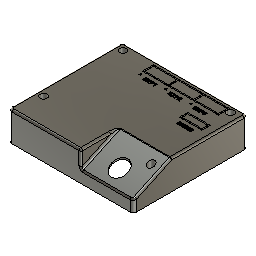
TFT35-E3-V3.0-case (Autodesk Fusion 360 design; units mm, degrees)
Autodesk Fusion 360 part; units mm, degrees
note: some values were not read from the file. Chosen so that the rebuilt part matches the saved one: which face or edge a step refers to; the layout of a text.
imported_body "Derived Base Feature1" makes body 1
move_body "Move1" bodies 1 to x (1, 0, 0) y (0, 0, 1) z (0, -1, 0) at (0, 0, 0)
sketch "mounting plate back" plane through (0, 0, 0) normal (0, 0, 1) x (-1, 0, 0)
  arc A0 (-83.1, -77.3055) -> (-80.1, -80.3055) centre (-80.1, -77.3055) ccw
  line L0 (-80.1, -80.3055) -> (15.9, -80.3055)
  arc A1 (15.9, -80.3055) -> (18.9, -77.3055) centre (15.9, -77.3055) ccw
  line L1 (18.9, -77.3055) -> (18.9, 33.4204)
  line L2 (18.9, 33.4204) -> (-83.1, 33.4204)
  line L3 (-83.1, 33.4204) -> (-83.1, -77.3055)
  line L4 (8.2, -16) -> (8.2, -68)
  line L5 (8.2, -68) -> (-71.6, -68)
  line L6 (-71.6, -68) -> (-71.6, -16)
  line L7 (-71.6, -16) -> (8.2, -16)
  circle A2 centre (0, 0) radius 5
  circle A3 centre (12.85, -9.55) radius 3
  circle A4 centre (12.85, -74.45) radius 3
  circle A5 centre (-75.05, -74.45) radius 3
  circle A6 centre (-75.05, -9.55) radius 3
  line L8 (18.9, 13) -> (-83.1, 13)
  line L9 (-83.1, 13) -> (-83.1, -80.2)
  line L10 (-83.1, -80.2) -> (18.9, -80.2)
  line L11 (18.9, -80.2) -> (18.9, 13)
  point P0 (12.85, -74.45)
  point P1 (-75.05, -74.45)
  point P2 (-75.05, -9.55)
  point P3 (12.85, -9.55)
  dimension "d5" = 93.2
  dimension "d6" = 102
  dimension "d7" = 13
  constraint coincident L1 L8.start
  constraint horizontal L8
  constraint vertical L9
  constraint horizontal L10
  constraint vertical L11
  constraint coincident P0 A4.centre
  constraint coincident P1 A5.centre
  constraint coincident P2 A6.centre
  constraint coincident P3 A3.centre
  constraint coincident A2.centre origin
  measures "d5" distance of L8.start L10.end
  measures "d6" distance of L8.start L8.end
  measures "d7" distance of L8 A2.centre
extrude "Extrude1" add sketch "mounting plate back" along normal blind 24 separate body contours A0 A1 L1 L3 L8 L9 L10 L11 | A0 L9 L10 | A1 L10 L11 | L4 L5 L6 L7 | A2 | A3 | A4 | A5 | A6 makes body 2
sketch "back box top" plane through (0, 0, 24) normal (0, 0, 1) x (-1, 0, 0)
  line L0 (18.9, -80.2) -> (18.9, 13)
  line L1 (18.9, 13) -> (-83.1, 13)
  line L2 (-83.1, 13) -> (-83.1, -80.2)
  line L3 (-83.1, -80.2) -> (18.9, -80.2)
  circle A0 centre (12.85, -74.45) radius 2.75
  circle A1 centre (-75.05, -74.45) radius 2.75
  circle A2 centre (12.85, -9.55) radius 2.75
  circle A3 centre (-75.05, -9.55) radius 2.75
  circle A4 centre (-59.9601, 1.1026) radius 6.75
  line L4 (-57.4705, -50.4562) -> (-75.7215, -50.4562)
  line L5 (-75.7215, -50.4562) -> (-75.7215, -57.1364)
  line L6 (-75.7215, -57.1364) -> (-57.4705, -57.1364)
  line L7 (-57.4705, -57.1364) -> (-57.4705, -50.4562)
  line L8 (-71.8313, -67.8197) -> (-9.744, -67.8197)
  line L9 (-9.744, -67.8197) -> (-9.744, -76.8684)
  line L10 (-9.744, -76.8684) -> (-71.8313, -76.8684)
  line L11 (-71.8313, -76.8684) -> (-71.8313, -67.8197)
  line L12 (-75.7215, -53.7963) -> (-57.4705, -53.7963) construction
  line L13 (-66.596, -50.4562) -> (-66.596, -57.1364) construction
  line L14 (-9.744, -72.3441) -> (-71.8313, -72.3441) construction
  line L15 (-74.7215, -56.1364) -> (-58.4705, -56.1364)
  line L16 (-58.4705, -56.1364) -> (-58.4705, -51.4562)
  line L17 (-58.4705, -51.4562) -> (-74.7215, -51.4562)
  line L18 (-74.7215, -51.4562) -> (-74.7215, -56.1364)
  line L19 (-65.596, -50.4562) -> (-67.596, -50.4562)
  line L20 (-67.596, -50.4562) -> (-67.596, -51.4562)
  line L21 (-65.596, -51.4562) -> (-65.596, -50.4562)
  line L22 (-57.4705, -54.7963) -> (-58.4705, -54.7963)
  line L23 (-58.4705, -52.7963) -> (-57.4705, -52.7963)
  line L24 (-57.4705, -52.7963) -> (-57.4705, -54.7963)
  line L25 (-67.596, -57.1364) -> (-65.596, -57.1364)
  line L26 (-65.596, -57.1364) -> (-65.596, -56.1364)
  line L27 (-67.596, -56.1364) -> (-67.596, -57.1364)
  line L28 (-75.7215, -54.7963) -> (-74.7215, -54.7963)
  line L29 (-74.7215, -52.7963) -> (-75.7215, -52.7963)
  line L30 (-75.7215, -52.7963) -> (-75.7215, -54.7963)
  line L31 (-70.8313, -75.8684) -> (-70.8313, -68.8197)
  line L32 (-10.744, -68.8197) -> (-10.744, -75.8684)
  line L33 (-71.8313, -73.3441) -> (-70.8313, -73.3441)
  line L34 (-70.8313, -71.3441) -> (-71.8313, -71.3441)
  line L35 (-71.8313, -71.3441) -> (-71.8313, -73.3441)
  line L36 (-9.744, -71.3441) -> (-10.744, -71.3441)
  line L37 (-10.744, -73.3441) -> (-9.744, -73.3441)
  line L38 (-9.744, -73.3441) -> (-9.744, -71.3441)
  line L39 (-40.7876, -76.8684) -> (-40.7876, -67.8197) construction
  line L40 (-39.7876, -67.8197) -> (-41.7876, -67.8197)
  line L41 (-41.7876, -67.8197) -> (-41.7876, -68.8197)
  line L42 (-39.7876, -68.8197) -> (-39.7876, -67.8197)
  line L43 (-41.7876, -76.8684) -> (-39.7876, -76.8684)
  line L44 (-39.7876, -76.8684) -> (-39.7876, -75.8684)
  line L45 (-41.7876, -75.8684) -> (-41.7876, -76.8684)
  line L46 (-30.4396, -67.8197) -> (-30.4396, -76.8684) construction
  line L47 (-51.1356, -67.8197) -> (-51.1356, -76.8684) construction
  line L48 (-29.9396, -68.8197) -> (-29.9396, -75.8684)
  line L49 (-30.9396, -75.8684) -> (-30.9396, -68.8197)
  line L50 (-29.9396, -68.8197) -> (-10.744, -68.8197)
  line L51 (-10.744, -75.8684) -> (-29.9396, -75.8684)
  line L52 (-30.9396, -73.3441) -> (-30.4396, -73.3441)
  line L53 (-20.3418, -68.8197) -> (-20.3418, -75.8684) construction
  line L54 (-19.3418, -67.8197) -> (-21.3418, -67.8197)
  line L55 (-21.3418, -67.8197) -> (-21.3418, -68.8197)
  line L56 (-19.3418, -68.8197) -> (-19.3418, -67.8197)
  line L57 (-21.3418, -76.8684) -> (-21.3418, -75.8684)
  line L58 (-19.3418, -75.8684) -> (-19.3418, -76.8684)
  line L59 (-50.6356, -75.8684) -> (-50.6356, -68.8197)
  line L60 (-51.6356, -68.8197) -> (-51.6356, -75.8684)
  line L61 (-70.8313, -68.8197) -> (-51.6356, -68.8197)
  line L62 (-50.6356, -68.8197) -> (-30.9396, -68.8197)
  line L63 (-30.9396, -75.8684) -> (-50.6356, -75.8684)
  line L64 (-51.6356, -75.8684) -> (-70.8313, -75.8684)
  line L65 (-51.6356, -73.3441) -> (-50.6356, -73.3441)
  line L66 (-50.6356, -73.3441) -> (-50.6356, -71.3441)
  line L67 (-50.6356, -71.3441) -> (-51.6356, -71.3441)
  line L68 (-51.6356, -71.3441) -> (-51.6356, -73.3441)
  line L69 (-61.2335, -68.8197) -> (-61.2335, -75.8684) construction
  line L70 (-60.2335, -67.8197) -> (-62.2335, -67.8197)
  line L71 (-62.2335, -67.8197) -> (-62.2335, -68.8197)
  line L72 (-60.2335, -68.8197) -> (-60.2335, -67.8197)
  line L73 (-62.2335, -76.8684) -> (-60.2335, -76.8684)
  line L74 (-60.2335, -76.8684) -> (-60.2335, -75.8684)
  line L75 (-62.2335, -75.8684) -> (-62.2335, -76.8684)
  line L76 (-30.9396, -73.3441) -> (-29.9396, -73.3441)
  line L77 (-29.9396, -73.3441) -> (-29.9396, -71.3441)
  line L78 (-29.9396, -71.3441) -> (-30.9396, -71.3441)
  line L79 (-30.9396, -71.3441) -> (-30.9396, -73.3441)
  line L80 (-30.9396, -73.3441) -> (-29.9396, -71.3441) construction
  line L81 (-29.9396, -73.3441) -> (-30.9396, -71.3441) construction
  line L82 (-52.2335, -76.8684) -> (-52.2335, -75.8684)
  line L83 (-54.2335, -75.8684) -> (-54.2335, -76.8684)
  line L84 (-54.2335, -76.8684) -> (-52.2335, -76.8684)
  line L85 (-68.2335, -76.8684) -> (-68.2335, -75.8684)
  line L86 (-70.2335, -75.8684) -> (-70.2335, -76.8684)
  line L87 (-70.2335, -76.8684) -> (-68.2335, -76.8684)
  line L88 (-54.2335, -67.8197) -> (-54.2335, -68.8197)
  line L89 (-52.2335, -67.8197) -> (-54.2335, -67.8197)
  line L90 (-52.2335, -68.8197) -> (-52.2335, -67.8197)
  line L91 (-70.2335, -67.8197) -> (-70.2335, -68.8197)
  line L92 (-68.2335, -67.8197) -> (-70.2335, -67.8197)
  line L93 (-68.2335, -68.8197) -> (-68.2335, -67.8197)
  line L94 (-33.7876, -76.8684) -> (-31.7876, -76.8684)
  line L95 (-31.7876, -76.8684) -> (-31.7876, -75.8684)
  line L96 (-33.7876, -75.8684) -> (-33.7876, -76.8684)
  line L97 (-49.7876, -76.8684) -> (-47.7876, -76.8684)
  line L98 (-47.7876, -76.8684) -> (-47.7876, -75.8684)
  line L99 (-49.7876, -75.8684) -> (-49.7876, -76.8684)
  line L100 (-31.7876, -68.8197) -> (-31.7876, -67.8197)
  line L101 (-31.7876, -67.8197) -> (-33.7876, -67.8197)
  line L102 (-33.7876, -67.8197) -> (-33.7876, -68.8197)
  line L103 (-47.7876, -68.8197) -> (-47.7876, -67.8197)
  line L104 (-47.7876, -67.8197) -> (-49.7876, -67.8197)
  line L105 (-49.7876, -67.8197) -> (-49.7876, -68.8197)
  line L106 (-11.3418, -68.8197) -> (-11.3418, -67.8197)
  line L107 (-11.3418, -67.8197) -> (-13.3418, -67.8197)
  line L108 (-13.3418, -67.8197) -> (-13.3418, -68.8197)
  line L109 (-27.3418, -68.8197) -> (-27.3418, -67.8197)
  line L110 (-27.3418, -67.8197) -> (-29.3418, -67.8197)
  line L111 (-29.3418, -67.8197) -> (-29.3418, -68.8197)
  line L112 (-21.3418, -76.8684) -> (-21.3418, -75.8684)
  line L113 (-19.3418, -75.8684) -> (-19.3418, -76.8684)
  line L114 (-11.3418, -75.8684) -> (-11.3418, -76.8684)
  line L115 (-11.3418, -75.8684) -> (-11.3418, -76.8684)
  line L116 (-13.3418, -76.8684) -> (-13.3418, -75.8684)
  line L117 (-13.3418, -76.8684) -> (-13.3418, -75.8684)
  line L118 (-27.3418, -75.8684) -> (-27.3418, -76.8684)
  line L119 (-27.3418, -75.8684) -> (-27.3418, -76.8684)
  line L120 (-29.3418, -76.8684) -> (-29.3418, -75.8684)
  line L121 (-29.3418, -76.8684) -> (-29.3418, -75.8684)
  line L122 (-61.096, -56.1364) -> (-61.096, -57.1364)
  line L123 (-59.096, -57.1364) -> (-59.096, -56.1364)
  line L124 (-61.096, -57.1364) -> (-59.096, -57.1364)
  line L125 (-73.996, -56.1364) -> (-73.996, -57.1364)
  line L126 (-71.996, -57.1364) -> (-71.996, -56.1364)
  line L127 (-73.996, -57.1364) -> (-71.996, -57.1364)
  line L128 (-72.096, -51.4562) -> (-72.096, -50.4562)
  line L129 (-74.096, -50.4562) -> (-74.096, -51.4562)
  line L130 (-72.096, -50.4562) -> (-74.096, -50.4562)
  line L131 (-59.096, -51.4562) -> (-59.096, -50.4562)
  line L132 (-61.096, -50.4562) -> (-61.096, -51.4562)
  line L133 (-59.096, -50.4562) -> (-61.096, -50.4562)
  line L134 (-9.9786, -61.8197) -> (-71.9086, -61.8197) construction
  line L135 (-57.8501, -44.4562) -> (-75.3418, -44.4562) construction
  line L136 (-66.596, -50.4562) -> (-66.596, -44.4562) construction
  line L137 (-61.2335, -68.8197) -> (-61.2335, -61.8197) construction
  line L138 (-40.7876, -68.8197) -> (-40.7876, -61.8197) construction
  line L139 (-20.3418, -68.8197) -> (-20.3418, -61.8197) construction
  line L140 (-15.6983, -61.8197) -> (-24.9854, -61.8197) construction
  line L141 (-24.9854, -61.8197) -> (-24.9854, -65.8197) construction
  line L142 (-24.9854, -65.8197) -> (-15.6983, -65.8197) construction
  line L143 (-15.6983, -65.8197) -> (-15.6983, -61.8197) construction
  line L144 (-35.9195, -61.8197) -> (-45.6558, -61.8197) construction
  line L145 (-45.6558, -61.8197) -> (-45.6558, -65.8197) construction
  line L146 (-45.6558, -65.8197) -> (-35.9195, -65.8197) construction
  line L147 (-35.9195, -65.8197) -> (-35.9195, -61.8197) construction
  line L148 (-56.3507, -61.8197) -> (-66.1163, -61.8197) construction
  line L149 (-66.1163, -61.8197) -> (-66.1163, -65.8197) construction
  line L150 (-66.1163, -65.8197) -> (-56.3507, -65.8197) construction
  line L151 (-56.3507, -65.8197) -> (-56.3507, -61.8197) construction
  line L152 (-60.7278, -44.4562) -> (-72.4642, -44.4562) construction
  line L153 (-72.4642, -44.4562) -> (-72.4642, -48.4562) construction
  line L154 (-72.4642, -48.4562) -> (-60.7278, -48.4562) construction
  line L155 (-60.7278, -48.4562) -> (-60.7278, -44.4562) construction
  line L156 (-12.2078, -64.0824) -> (-11.3418, -65.5824)
  line L157 (-11.3418, -65.5824) -> (-10.4758, -64.0824)
  line L158 (-10.4758, -64.0824) -> (-12.2078, -64.0824)
  line L159 (-12.2078, -64.0824) -> (-11.3418, -65.5824)
  line L160 (-11.3418, -65.5824) -> (-10.4758, -64.0824)
  line L161 (-10.4758, -64.0824) -> (-12.2078, -64.0824)
  line L162 (-32.9038, -64.0824) -> (-32.0378, -65.5824)
  line L163 (-32.0378, -65.5824) -> (-31.1718, -64.0824)
  line L164 (-32.9038, -64.0824) -> (-32.0378, -65.5824)
  line L165 (-31.1718, -64.0824) -> (-32.9038, -64.0824)
  line L166 (-32.0378, -65.5824) -> (-31.1718, -64.0824)
  line L167 (-31.1718, -64.0824) -> (-32.9038, -64.0824)
  line L168 (-53.5998, -64.0824) -> (-52.7338, -65.5824)
  line L169 (-51.8678, -64.0824) -> (-53.5998, -64.0824)
  line L170 (-53.5998, -64.0824) -> (-52.7338, -65.5824)
  line L171 (-51.8678, -64.0824) -> (-53.5998, -64.0824)
  line L172 (-52.7338, -65.5824) -> (-51.8678, -64.0824)
  line L173 (-52.7338, -65.5824) -> (-51.8678, -64.0824)
  point P0 (12.85, -74.45)
  point P1 (-75.05, -74.45)
  point P2 (-75.05, -9.55)
  point P3 (12.85, -9.55)
  point P4 (-30.4396, -72.3441)
  point P5 (-20.3418, -68.8197)
  point P6 (-20.3418, -75.8684)
  point P7 (-51.1356, -72.3441)
  point P8 (-61.2335, -68.8197)
  point P9 (-61.2335, -75.8684)
  point P10 (-30.4396, -72.3441)
  point P11 (-53.2335, -75.8684)
  point P12 (-53.2335, -75.8684)
  point P13 (-69.2335, -75.8684)
  point P14 (-69.2335, -75.8684)
  point P15 (-53.2335, -68.8197)
  point P16 (-53.2335, -68.8197)
  point P17 (-69.2335, -68.8197)
  point P18 (-69.2335, -68.8197)
  point P19 (-32.7876, -76.8684)
  point P20 (-48.7876, -76.8684)
  point P21 (-32.7876, -67.8197)
  point P22 (-48.7876, -67.8197)
  point P23 (-12.3418, -68.8197)
  point P24 (-12.3418, -68.8197)
  point P25 (-28.3418, -68.8197)
  point P26 (-28.3418, -68.8197)
  point P27 (-20.3418, -75.8684)
  point P28 (-20.3418, -75.8684)
  point P29 (-12.3418, -75.8684)
  point P30 (-12.3418, -75.8684)
  point P31 (-12.3418, -75.8684)
  point P32 (-12.3418, -75.8684)
  point P33 (-28.3418, -75.8684)
  point P34 (-28.3418, -75.8684)
  point P35 (-28.3418, -75.8684)
  point P36 (-28.3418, -75.8684)
  point P37 (-60.096, -57.1364)
  point P38 (-72.996, -57.1364)
  point P39 (-73.096, -50.4562)
  point P40 (-60.096, -50.4562)
  point P41 (-11.3418, -64.5824)
  point P42 (-11.3418, -64.5824)
  point P43 (-32.0378, -64.5824)
  point P44 (-32.0378, -64.5824)
  point P45 (-52.7338, -64.5824)
  point P46 (-52.7338, -64.5824)
  dimension "d21" = 5.5
  dimension "d22" = 5.5
  dimension "d23" = 5.5
  dimension "d24" = 5.5
  dimension "d37" = 13.5
  dimension "d101" = -1
  dimension "d118" = 20.6957
  dimension "d119" = 20.6957
  dimension "d120" = 1
  dimension "d125" = 1
  dimension "d126" = 2
  dimension "d141" = 6
  dimension "d142" = 6
  dimension "d146" = 0.5
  dimension "d147" = 0.5
  dimension "d148" = 0.5
  dimension "d149" = 0.5
  dimension "d150" = 0.5
  dimension "d151" = 0.5
  text T0 "EXP1" font "Arial" height 4 bold align ink ink in box 0 x 0 at (-15.7083, -61.8397) x (-1, 0) y (0, -1) spacing 1 height is em
  text T1 "EXP2" font "Arial" height 4 bold align ink ink in box 0 x 0 at (-35.9295, -61.8397) x (-1, 0) y (0, -1) spacing 1 height is em
  text T2 "EXP3" font "Arial" height 4 bold align ink ink in box 0 x 0 at (-56.3607, -61.8397) x (-1, 0) y (0, -1) spacing 1 height is em
  text T3 "RS232" font "Arial" height 4 bold align ink ink in box 0 x 0 at (-60.7378, -44.4762) x (-1, 0) y (0, -1) spacing 1 height is em
  constraint coincident P0 A0.centre
  constraint coincident P1 A1.centre
  constraint coincident P3 A2.centre
  constraint coincident P2 A3.centre
  constraint midpoint L4 L13.start
  constraint perpendicular L19 L20
  constraint parallel L20 L21
  constraint horizontal L19
  constraint coincident L4 L19.start
  constraint parallel L22 L23
  constraint horizontal L22
  constraint perpendicular L25 L26
  constraint parallel L26 L27
  constraint horizontal L25
  constraint parallel L28 L29
  constraint horizontal L28
  constraint parallel L33 L34
  constraint horizontal L33
  constraint parallel L36 L37
  constraint horizontal L36
  constraint parallel L11 L31
  constraint parallel L8 L61
  constraint parallel L9 L32
  constraint perpendicular L40 L41
  constraint parallel L41 L42
  constraint horizontal L40
  constraint perpendicular L43 L44
  constraint parallel L44 L45
  constraint horizontal L43
  constraint coincident L8 L46.start
  constraint coincident L10 L46.end
  constraint perpendicular L10 L46
  constraint coincident L8 L47.start
  constraint coincident L10 L47.end
  constraint perpendicular L10 L47
  constraint parallel L48 L49
  constraint collinear L50 L61
  constraint collinear L51 L63
  constraint horizontal L52
  constraint midpoint L50 P5
  constraint midpoint L51 P28
  constraint perpendicular L51 L53
  constraint perpendicular L54 L55
  constraint parallel L55 L56
  constraint horizontal L54
  constraint coincident P5 L53.start
  constraint parallel L57 L58
  constraint coincident P28 P27
  constraint parallel L59 L60
  constraint collinear L61 L62
  constraint collinear L63 L64
  constraint perpendicular L65 L66
  constraint parallel L65 L67
  constraint parallel L66 L68
  constraint horizontal L65
  constraint midpoint L61 P8
  constraint midpoint L64 P9
  constraint perpendicular L64 L69
  constraint perpendicular L70 L71
  constraint parallel L71 L72
  constraint horizontal L70
  constraint coincident P8 L69.start
  constraint perpendicular L73 L74
  constraint parallel L74 L75
  constraint horizontal L73
  constraint coincident P9 L69.end
  constraint coincident L64 L74.end
  constraint coincident L64 L75.start
  constraint coincident L31 L33.end
  constraint coincident L31 L34.start
  constraint coincident L61 L71.end
  constraint coincident L61 L72.start
  constraint coincident L63 L45.start
  constraint coincident L63 L44.end
  constraint coincident L62 L41.end
  constraint coincident L62 L42.start
  constraint coincident L49 L52.start
  constraint coincident L46 L52.end
  constraint perpendicular L76 L77
  constraint parallel L76 L78
  constraint parallel L77 L79
  constraint horizontal L76
  constraint coincident L80 P10
  constraint coincident L81 P10
  constraint coincident P10 P4
  constraint coincident L50 L56.start
  constraint coincident L50 L55.end
  constraint coincident L51 L58.start
  constraint coincident L51 L57.end
  constraint coincident L10 L57.start
  constraint coincident L10 L58.end
  constraint coincident L32 L37.start
  constraint coincident L32 L36.end
  constraint coincident L18 L29.start
  constraint coincident L18 L28.end
  constraint coincident L15 L27.start
  constraint coincident L15 L26.end
  constraint coincident L17 L20.end
  constraint coincident L17 L21.start
  constraint coincident L16 L23.start
  constraint coincident L16 L22.end
  constraint perpendicular L82 L84
  constraint parallel L82 L83
  constraint horizontal L84
  constraint coincident P12 P11
  constraint perpendicular L85 L87
  constraint parallel L85 L86
  constraint horizontal L87
  constraint coincident P14 P13
  constraint perpendicular L88 L89
  constraint parallel L88 L90
  constraint horizontal L89
  constraint coincident P16 P15
  constraint perpendicular L91 L92
  constraint parallel L91 L93
  constraint horizontal L92
  constraint coincident P18 P17
  constraint perpendicular L94 L95
  constraint parallel L95 L96
  constraint horizontal L94
  constraint perpendicular L97 L98
  constraint parallel L98 L99
  constraint horizontal L97
  constraint perpendicular L101 L102
  constraint parallel L100 L102
  constraint horizontal L101
  constraint perpendicular L104 L105
  constraint parallel L103 L105
  constraint horizontal L104
  constraint perpendicular L107 L108
  constraint parallel L106 L108
  constraint horizontal L107
  constraint coincident P24 P23
  constraint perpendicular L110 L111
  constraint parallel L109 L111
  constraint horizontal L110
  constraint coincident P26 P25
  constraint parallel L112 L113
  constraint parallel L114 L117
  constraint coincident P32 P31
  constraint parallel L115 L116
  constraint parallel L118 L121
  constraint coincident P36 P35
  constraint parallel L119 L120
  constraint perpendicular L123 L124
  constraint parallel L122 L123
  constraint horizontal L124
  constraint perpendicular L126 L127
  constraint parallel L125 L126
  constraint horizontal L127
  constraint perpendicular L129 L130
  constraint parallel L128 L129
  constraint horizontal L130
  constraint perpendicular L132 L133
  constraint parallel L131 L132
  constraint horizontal L133
  constraint horizontal L134
  constraint perpendicular L131 L135
  constraint midpoint L135 L136.end
  constraint vertical L13
  constraint vertical L136
  constraint coincident L134 L137.end
  constraint perpendicular L134 L137
  constraint midpoint L62 L138.start
  constraint coincident L134 L138.end
  constraint perpendicular L134 L138
  constraint coincident L134 L139.end
  constraint perpendicular L134 L139
  constraint perpendicular L140 L141
  constraint parallel L140 L142
  constraint parallel L141 L143
  constraint perpendicular L144 L145
  constraint parallel L144 L146
  constraint parallel L145 L147
  constraint midpoint L138.end L144
  constraint perpendicular L148 L149
  constraint parallel L148 L150
  constraint parallel L149 L151
  constraint perpendicular L152 L153
  constraint parallel L152 L154
  constraint parallel L153 L155
  measures "d21" diameter of A0
  measures "d22" diameter of A1
  measures "d23" diameter of A2
  measures "d24" diameter of A3
  measures "d37" diameter of A4
  measures "d118" distance of L9 L46
  measures "d119" distance of L11 L47
  measures "d120" distance of L48.end L49.start
  measures "d125" distance of L59.end L60.start
  measures "d126" distance of L65.end L66.end
  measures "d141" distance of L8 L134
  measures "d142" distance of L4 L135
  measures "d146" distance of P42 L158
  measures "d147" distance of P42 L161
  measures "d148" distance of P44 L167
  measures "d149" distance of P44 L165
  measures "d150" distance of P46 L169
  measures "d151" distance of P46 L171
sketch "inside bracket face" plane through (0, -27.4513, -12.8008) normal (0, 0.906308, 0.422618) x (-1, 0, 0)
  arc A0 (-80.1, 57.1241) -> (-83.1, 54.1241) centre (-80.1, 54.1241) ccw
  line L0 (-83.1, 54.1241) -> (-83.1, 14.1241)
  line L1 (-83.1, 14.1241) -> (18.9, 14.1241)
  line L2 (18.9, 14.1241) -> (18.9, 54.1241)
  arc A1 (18.9, 54.1241) -> (15.9, 57.1241) centre (15.9, 54.1241) ccw
  line L3 (15.9, 57.1241) -> (-80.1, 57.1241)
  circle A2 centre (-73.1, 48.1241) radius 2.8
  circle A3 centre (-53.1, 28.1241) radius 2.8
  line L4 (-83.1, 14.1241) -> (-40.1, 14.1241)
  line L5 (-40.1, 14.1241) -> (-40.1, 57.1241)
  line L6 (-40.1, 57.1241) -> (-83.1, 57.1241)
  line L7 (-83.1, 57.1241) -> (-83.1, 14.1241)
  dimension "d28" = 43
  constraint horizontal L4
  constraint vertical L5
  constraint horizontal L6
  constraint vertical L7
  constraint coincident L0.end L1.start
  measures "d28" distance of L0.end L4.end
extrude "Extrude4" cut sketch "inside bracket face" along normal blind 120 contours A0 L0 L1 L3 L4 L5 L6 L7 | A0 L6 L7 | A2 | A3 bodies 2
extrude "Extrude3" cut sketch "back box top" against normal blind 12.75 contours A0 | A1 | A2 | A3 bodies 2
move_face "OffsetFaces2" offset -0.1 4 faces at (-15.5966, 9.6871, 15.5) (-15.515, 75.1286, 15.5) (72.385, 75.1286, 15.5) (72.3035, 9.4105, 17.0435) on bodies 2
fillet "Fillet2" radius 2.75 4 edges at (-18.9, 80.2, 12) (83.1, 80.2, 12) (83.1, -13, 4.7611) (-18.9, -13, 12) on bodies 2
fillet "Fillet2" radius 1.5 10 edges at (83.1, 49.1239, 24) (61.6, 18.0478, 24) (83.1, 2.5239, 16.7611) (40.1, 2.5239, 16.7611) (40.1, 2.5239, 24) (40.1, -13, 16.7611) (10.6, -13, 24) (61.6, -13, 9.5222) (-18.9, 33.6, 24) (32.1, 80.2, 24) on bodies 2
shell "Shell2" thickness 1.25 removed faces 1 at (16.0167, 49.1333, 0) on bodies 2
hole "Hole1" at (-12.85, 74.45, 24) at (75.05, 74.45, 24) at (75.05, 9.55, 24) at (-12.85, 9.55, 24) direction (0, 0, -1) diameter 3.2 depth 15 tip angle 180 bodies 2
sketch "inside back box" plane through (0, 0, 22.75) normal (0, 0, -1) x (1, 0, 0)
  ellipse E0 centre (41.6, -11.2817) end of major axis (41.6, -18.3803) minor radius 3 (38.6, -11.2817) -> (41.6, -18.3803) ccw
  line L0 (38.6, -11.2817) -> (38.6, 11.5)
  line L1 (38.6, 11.5) -> (-16.15, 11.5)
  arc A0 (-16.15, 11.5) -> (-17.4, 10.25) centre (-16.15, 10.25) ccw
  line L2 (-17.4, 10.25) -> (-17.4, -77.45)
  arc A1 (-17.4, -77.45) -> (-16.15, -78.7) centre (-16.15, -77.45) ccw
  line L3 (-16.15, -78.7) -> (80.35, -78.7)
  arc A2 (80.35, -78.7) -> (81.6, -77.45) centre (80.35, -77.45) ccw
  line L4 (81.6, -77.45) -> (81.6, -18.3803)
  line L5 (81.6, -18.3803) -> (41.6, -18.3803)
  circle A3 centre (-12.85, -9.55) radius 4.1
  circle A4 centre (75.05, -74.45) radius 4.1
  circle A5 centre (-12.85, -74.45) radius 4.1
  line L6 (-16.15, 10.25) -> (23.85, 10.25)
  line L7 (23.85, 10.25) -> (23.85, -8.75)
  line L8 (23.85, -8.75) -> (-16.15, -8.75)
  line L9 (-16.15, -8.75) -> (-16.15, 10.25)
  dimension "d156" = 1.25
  dimension "d157" = 40
  dimension "d158" = 19
  constraint horizontal L6
  constraint vertical L7
  constraint horizontal L8
  constraint vertical L9
  constraint coincident A0.centre L6.start
  measures "d156" distance of L2 L9
  measures "d157" distance of L7 L9
  measures "d158" distance of L6 L8
extrude "Extrude19" cut sketch "inside back box" against normal blind 0.5 contours A3 L6 L7 L8 L9 bodies 2
sketch "slot face" plane through (-18.9, 0, 0) normal (-1, 0, 0) x (0, -1, 0)
  line L0 (10.25, 0) -> (10.25, 22.5)
  line L1 (10.25, 22.5) -> (-77.45, 22.5)
  line L2 (-77.45, 22.5) -> (-77.45, 0)
  line L3 (-77.45, 0) -> (10.25, 0)
  line L4 (-62.9757, 11) -> (-30.0763, 11) construction
  line L5 (-27.9791, 14) -> (-10.8084, 14) construction
  line L6 (-27.3286, 27.9844) -> (-27.3286, -7.3526) construction
  line L7 (-14.3909, 27.9677) -> (-14.3909, -4.2878) construction
  line L8 (-31.9117, 30.3251) -> (-31.9117, -10.3251) construction
  line L9 (-58.8063, 30.5503) -> (-58.8063, -9.8701) construction
  line L10 (-58.8063, 11) -> (-31.9117, 11) construction
  line L11 (-27.3286, 14) -> (-14.3909, 14) construction
  line L12 (-58.8063, 14.5) -> (-31.9117, 14.5)
  line L13 (-31.9117, 14.5) -> (-31.9117, 10)
  line L14 (-31.9117, 10) -> (-58.8063, 10)
  line L15 (-58.8063, 10) -> (-58.8063, 14.5)
  line L16 (-27.3286, 18.5) -> (-14.3909, 18.5)
  line L17 (-14.3909, 18.5) -> (-14.3909, 10.5)
  line L18 (-14.3909, 10.5) -> (-27.3286, 10.5)
  line L19 (-27.3286, 10.5) -> (-27.3286, 18.5)
  dimension "d137" = 10
  dimension "d138" = 14.5
  dimension "d139" = 10.5
  dimension "d140" = 18.5
  constraint parallel L3 L4
  constraint parallel L3 L5
  constraint perpendicular L3 L6
  constraint perpendicular L1 L7
  constraint perpendicular L1 L8
  constraint perpendicular L1 L9
  constraint coincident L8 L10.end
  constraint coincident L4 L10.end
  constraint perpendicular L8 L10
  constraint coincident L9 L10.start
  constraint coincident L5 L11.end
  constraint coincident L7 L11.end
  constraint perpendicular L7 L11
  constraint coincident L6 L11.start
  constraint horizontal L12
  constraint vertical L13
  constraint horizontal L14
  constraint vertical L15
  constraint midpoint L8 L13.end
  constraint coincident L9 L12.start
  constraint horizontal L16
  constraint vertical L17
  constraint horizontal L18
  constraint vertical L19
  constraint coincident L7 L17.end
  constraint coincident L6 L16.start
  measures "d137" distance of L3 L14
  measures "d138" distance of L3 L12
  measures "d139" distance of L3 L18
  measures "d140" distance of L3 L16
extrude "Extrude14" cut sketch "slot face" against normal up to surface (1.25 mm away) contours L12 L13 L14 L15 | L16 L17 L18 L19 bodies 2
extrude "Extrude15" cut sketch "back box top" against normal blind 20 contours A4 | L4 L7 L16 L17 L23 L131 | L4 L17 L131 L132 L133 | L7 L16 L22 L23 L24 | L4 L17 L21 L132 | L15 L16 L17 L18 | L6 L7 L15 L16 L22 L123 | L4 L17 L19 L20 L21 | L4 L17 L20 L128 | L6 L15 L122 L123 L124 | L4 L17 L128 L129 L130 | L6 L15 L26 L122 | L4 L5 L17 L18 L29 L129 | L6 L15 L25 L26 L27 | L6 L15 L27 L126 | L5 L18 L28 L29 L30 | L6 L15 L125 L126 L127 | L5 L6 L15 L18 L28 L125 | L8 L11 L31 L34 L61 L91 | L8 L61 L91 L92 L93 | L11 L31 L33 L34 L35 | L8 L61 L71 L93 | L31 L60 L61 L64 L68 | L10 L11 L31 L33 L64 L86 | L8 L61 L70 L71 L72 | L8 L61 L72 L88 | L10 L64 L85 L86 L87 | L8 L61 L88 L89 L90 | L10 L64 L75 L85 | L8 L59 L60 L61 L62 L67 L90 L105 | L10 L64 L73 L74 L75 | L8 L62 L103 L104 L105 | L10 L64 L74 L83 | L8 L41 L62 L103 | L49 L59 L62 L63 L66 L79 | L10 L64 L82 L83 L84 | L8 L40 L41 L42 L62 | L59 L60 L65 L66 L67 L68 | L10 L59 L60 L63 L64 L65 L82 L99 | L8 L42 L62 L102 | L10 L63 L97 L98 L99 | L8 L62 L100 L101 L102 | L10 L45 L63 L98 | L8 L48 L49 L50 L62 L78 L100 L111 | L10 L43 L44 L45 L63 | L8 L50 L109 L110 L111 | L10 L44 L63 L96 | L8 L50 L55 L109 | L32 L48 L50 L51 L77 | L10 L63 L94 L95 L96 | L8 L50 L54 L55 L56 | L48 L49 L52 L76 L77 L78 L79 | L10 L48 L49 L51 L52 L63 L76 L95 L120 L121 | L8 L50 L56 L108 | L10 L51 L118 L119 L120 L121 | L8 L50 L106 L107 L108 | L10 L51 L57 L112 L118 L119 | L8 L9 L32 L36 L50 L106 | L10 L51 L57 L58 L112 L113 | L10 L51 L58 L113 L116 L117 | L9 L32 L36 L37 L38 | L10 L51 L114 L115 L116 L117 | L9 L10 L32 L37 L51 L114 L115 bodies 2
extrude "Extrude16" add sketch "back box top" against normal blind 1 separate body contours L15 L16 L17 L18 | L31 L60 L61 L64 L68 | L49 L59 L62 L63 L66 L79 | L32 L48 L50 L51 L77 makes body 3 at (44.0703, 71.1693, 24) makes body 4 at (64.4327, 71.1693, 24) makes body 5 at (23.5411, 71.1693, 24) makes body 6 at (69.3045, 54.5763, 24)
extrude "Extrude17" add sketch "back box top" against normal blind 0.25 contours L4 L17 L131 L132 L133 | L7 L16 L22 L23 L24 | L4 L17 L19 L20 L21 | L6 L15 L122 L123 L124 | L4 L17 L128 L129 L130 | L6 L15 L25 L26 L27 | L5 L18 L28 L29 L30 | L6 L15 L125 L126 L127 | L8 L61 L91 L92 L93 | L11 L31 L33 L34 L35 | L8 L61 L70 L71 L72 | L10 L64 L85 L86 L87 | L8 L61 L88 L89 L90 | L10 L64 L73 L74 L75 | L8 L62 L103 L104 L105 | L10 L64 L82 L83 L84 | L8 L40 L41 L42 L62 | L59 L60 L65 L66 L67 L68 | L10 L63 L97 L98 L99 | L8 L62 L100 L101 L102 | L10 L43 L44 L45 L63 | L8 L50 L109 L110 L111 | L10 L63 L94 L95 L96 | L8 L50 L54 L55 L56 | L48 L49 L52 L76 L77 L78 L79 | L10 L51 L118 L119 L120 L121 | L8 L50 L106 L107 L108 | L10 L51 L57 L58 L112 L113 | L9 L32 L36 L37 L38 | L10 L51 L114 L115 L116 L117 bodies 2 3 4 5 6
extrude "Extrude18" cut sketch "back box top" sketch "back box top" against normal blind 0.5 contours L156 L157 L158 L159 L160 L161 | L162 L163 L164 L165 L166 L167 | L168 L169 L170 L171 L172 L173 of sketch 2 text T0 T1 T2 T3 bodies 2
hidden bodies 1
equation "d118 = ( 62.087 / 3 ) * 1 mm"
equation "d119 = ( 62.087 / 3 ) * 1 mm"
named bodies: "mounting plate", "back box"
